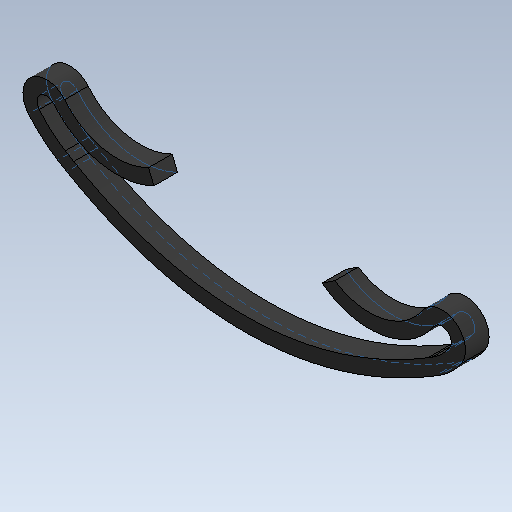
# Autodesk Inventor part: 脚ゴム
Saved by Autodesk Inventor 2020 (Build 240168000, 168)
## iProperties
Created: 2020-11-29
Part Number: 脚ゴム
Material: ゴム、黒
Document SubType Name: Modeling
Designer: AA19065
Density: 0.93 g/cm^3
Appearance: ゴム - 黒
Mass: 2.30491 g
Surface Area: 26.747 cm^2
Volume: 2.47839 cm^3
Author: AA19065
Autodesk Inventor part; units mm, degrees
ref_plane "YZ Plane" through (0, 0, 0) normal (1, 0, 0) x (0, 1, 0)
ref_plane "XZ Plane" through (0, 0, 0) normal (0, 1, 0) x (-1, 0, 0)
ref_plane "XY Plane" through (0, 0, 0) normal (0, 0, 1) x (1, 0, 0)
sketch "スケッチ1" plane through (0, 0, 0) normal (0, 0, 1) x (1, 0, 0)
  spline S0 degree 4 poles (38.5164, -45.3071) (32.8487, -48.7376) (24.871, -52.6644) (14.1977, -56.036) (0.8351, -57.2731) (-12.4819, -56.5781) (-23.1394, -53.6461) (-31.0456, -50.0372) (-36.604, -46.8264) knots 0 0 0 0 0 0.316482 0.440352 0.563601 0.687002 1 1 1 1 1
  circle A0 centre (0, 0) radius 1.3
  circle A1 centre (0, 0) radius 2.5
  circle A2 centre (0, 0) radius 5
  line L0 (4.899, 1) -> (9.798, -23)
  line L1 (-4.899, 1) -> (-9.798, -23)
  line L2 (-3.817, -10.1196) -> (-8.9705, -20.5808)
  circle A3 centre (0, -12) radius 4.255
  line L3 (3.817, -10.1196) -> (8.9705, -20.5808)
  circle A4 centre (0.0033, -24.9496) radius 10
  circle A5 centre (0, -25) radius 7.025
  spline S1 degree 4 poles (51.4895, -34.9586) (51.1529, -35.2256) (50.6846, -35.5944) (50.0873, -36.0604) (49.3638, -36.6179) (48.8453, -37.0139) (48.332, -37.4027) (47.8236, -37.7843) (47.3201, -38.159) (46.8211, -38.527) (46.3265, -38.8884) (45.8362, -39.2435) (45.3499, -39.5924) (44.8675, -39.9354) (44.3888, -40.2724) (43.9136, -40.6038) (43.4419, -40.9296) (42.9735, -41.25) (42.5081, -41.5651) (42.0458, -41.8751) (41.5864, -42.18) (41.1297, -42.48) (40.6756, -42.7752) (40.2241, -43.0657) (39.7749, -43.3517) (39.328, -43.6331) (38.8834, -43.9101) (38.4408, -44.1828) (38.0002, -44.4513) (37.5615, -44.7157) (37.1246, -44.9759) (36.6894, -45.2322) (36.2559, -45.4846) (35.8239, -45.7332) (35.3934, -45.9779) (34.9643, -46.2189) (34.5365, -46.4563) (34.1101, -46.6901) (33.6848, -46.9203) (33.2606, -47.1471) (32.8375, -47.3704) (32.4155, -47.5903) (31.9943, -47.8068) (31.5741, -48.0201) (31.1548, -48.23) (30.7362, -48.4368) (30.3184, -48.6403) (29.9013, -48.8407) (29.4848, -49.038) (29.069, -49.2322) (28.6537, -49.4233) (28.239, -49.6114) (27.8248, -49.7965) (27.411, -49.9786) (26.9977, -50.1578) (26.5847, -50.334) (26.1721, -50.5073) (25.7598, -50.6777) (25.3479, -50.8453) (24.9362, -51.01) (24.5247, -51.1719) (24.1135, -51.331) (23.7024, -51.4873) (23.2916, -51.6408) (22.8809, -51.7915) (22.4703, -51.9394) (22.0598, -52.0847) (21.6495, -52.2271) (21.2392, -52.3669) (20.829, -52.504) (20.4188, -52.6383) (20.0086, -52.77) (19.5985, -52.8989) (19.1884, -53.0252) (18.7783, -53.1489) (18.3681, -53.2698) (17.958, -53.3881) (17.5477, -53.5038) (17.1375, -53.6167) (16.7272, -53.7271) (16.3168, -53.8348) (15.9064, -53.9399) (15.4959, -54.0424) (15.0853, -54.1422) (14.6747, -54.2394) (14.2639, -54.334) (13.8531, -54.426) (13.4422, -54.5153) (13.0311, -54.6021) (12.62, -54.6862) (12.2088, -54.7677) (11.7975, -54.8466) (11.3861, -54.9229) (10.9746, -54.9966) (10.563, -55.0677) (10.1513, -55.1362) (9.7395, -55.2021) (9.3276, -55.2654) (8.9156, -55.3261) (8.5036, -55.3842) (8.0914, -55.4397) (7.6792, -55.4926) (7.2669, -55.5428) (6.8545, -55.5905) (6.4421, -55.6356) (6.0295, -55.6781) (5.617, -55.718) (5.2043, -55.7553) (4.7916, -55.79) (4.3789, -55.822) (3.9661, -55.8515) (3.5533, -55.8784) (3.1405, -55.9027) (2.7276, -55.9244) (2.3147, -55.9435) (1.9018, -55.96) (1.489, -55.9739) (1.0761, -55.9851) (0.6632, -55.9938) (0.2503, -55.9999) (-0.1625, -56.0034) (-0.5753, -56.0043) (-0.9881, -56.0026) (-1.4008, -55.9982) (-1.8134, -55.9913) (-2.2261, -55.9818) (-2.6386, -55.9697) (-3.0511, -55.955) (-3.4634, -55.9376) (-3.8757, -55.9177) (-4.2879, -55.8952) (-4.7, -55.8701) (-5.112, -55.8424) (-5.5239, -55.8121) (-5.9357, -55.7791) (-6.3473, -55.7436) (-6.7588, -55.7055) (-7.1701, -55.6648) (-7.5813, -55.6215) (-7.9923, -55.5756) (-8.4032, -55.5271) (-8.8139, -55.4761) (-9.2244, -55.4224) (-9.6348, -55.3661) (-10.0449, -55.3072) (-10.4549, -55.2458) (-10.8647, -55.1817) (-11.2743, -55.1151) (-11.6837, -55.0458) (-12.0928, -54.974) (-12.5018, -54.8995) (-12.9105, -54.8225) (-13.3191, -54.7429) (-13.7274, -54.6607) (-14.1355, -54.5759) (-14.5434, -54.4884) (-14.951, -54.3984) (-15.3585, -54.3058) (-15.7657, -54.2106) (-16.1727, -54.1128) (-16.5794, -54.0124) (-16.986, -53.9094) (-17.3923, -53.8038) (-17.7984, -53.6956) (-18.2043, -53.5848) (-18.61, -53.4713) (-19.0155, -53.3553) (-19.4208, -53.2366) (-19.8259, -53.1153) (-20.2308, -52.9913) (-20.6356, -52.8648) (-21.0401, -52.7355) (-21.4446, -52.6037) (-21.8489, -52.4692) (-22.253, -52.332) (-22.657, -52.1921) (-23.0609, -52.0496) (-23.4648, -51.9044) (-23.8685, -51.7565) (-24.2722, -51.6059) (-24.6759, -51.4526) (-25.0796, -51.2965) (-25.4832, -51.1377) (-25.8869, -50.9761) (-26.2907, -50.8117) (-26.6945, -50.6446) (-27.0985, -50.4746) (-27.5026, -50.3018) (-27.9068, -50.1261) (-28.3113, -49.9476) (-28.7161, -49.7661) (-29.1211, -49.5817) (-29.5265, -49.3944) (-29.9322, -49.204) (-30.3384, -49.0107) (-30.7451, -48.8142) (-31.1523, -48.6147) (-31.5601, -48.412) (-31.9685, -48.2062) (-32.3777, -47.9971) (-32.7876, -47.7847) (-33.1984, -47.569) (-33.6102, -47.3499) (-34.023, -47.1273) (-34.4368, -46.9012) (-34.8519, -46.6716) (-35.2682, -46.4382) (-35.686, -46.2011) (-36.1052, -45.9602) (-36.5261, -45.7154) (-36.9487, -45.4665) (-37.3732, -45.2135) (-37.7997, -44.9563) (-38.2284, -44.6947) (-38.6594, -44.4287) (-39.0929, -44.158) (-39.5291, -43.8825) (-39.9681, -43.6021) (-40.4101, -43.3165) (-40.8555, -43.0257) (-41.3043, -42.7295) (-41.7569, -42.4275) (-42.2135, -42.1196) (-42.6743, -41.8055) (-43.1398, -41.485) (-43.6102, -41.1578) (-44.0858, -40.8236) (-44.567, -40.482) (-45.0542, -40.1327) (-45.5479, -39.7753) (-46.0484, -39.4095) (-46.5564, -39.0347) (-47.0722, -38.6504) (-47.5966, -38.2562) (-48.13, -37.8515) (-48.6732, -37.4356) (-49.2269, -37.0078) (-50.01, -36.3976) (-50.6631, -35.8819) (-51.1798, -35.4699) (-51.5542, -35.1694) knots 0 0 0 0 0 0.01253 0.017489 0.022414 0.027307 0.032168 0.036998 0.041798 0.046569 0.051311 0.056026 0.060715 0.065378 0.070016 0.074629 0.079219 0.083786 0.088331 0.092854 0.097357 0.101839 0.106302 0.110746 0.115172 0.119579 0.12397 0.128343 0.132701 0.137042 0.141369 0.14568 0.149978 0.154261 0.158531 0.162788 0.167033 0.171265 0.175486 0.179695 0.183893 0.18808 0.192257 0.196424 0.200581 0.204729 0.208867 0.212997 0.217119 0.221232 0.225337 0.229434 0.233524 0.237607 0.241682 0.245751 0.249814 0.25387 0.25792 0.261964 0.266002 0.270035 0.274062 0.278085 0.282102 0.286114 0.290122 0.294125 0.298124 0.302119 0.30611 0.310097 0.31408 0.318059 0.322035 0.326007 0.329976 0.333942 0.337905 0.341865 0.345823 0.349777 0.353729 0.357678 0.361625 0.365569 0.369511 0.373451 0.377389 0.381325 0.385259 0.389191 0.393122 0.39705 0.400977 0.404903 0.408826 0.412749 0.41667 0.42059 0.424508 0.428426 0.432342 0.436257 0.440171 0.444085 0.447997 0.451908 0.455819 0.459729 0.463638 0.467547 0.471454 0.475362 0.479269 0.483175 0.487081 0.490987 0.494892 0.498797 0.502702 0.506607 0.510511 0.514415 0.51832 0.522224 0.526128 0.530033 0.533937 0.537842 0.541747 0.545652 0.549557 0.553463 0.557369 0.561276 0.565183 0.56909 0.572998 0.576907 0.580817 0.584727 0.588638 0.592549 0.596462 0.600375 0.60429 0.608205 0.612122 0.616039 0.619958 0.623879 0.6278 0.631723 0.635647 0.639573 0.643501 0.64743 0.651361 0.655294 0.659229 0.663165 0.667104 0.671045 0.674989 0.678934 0.682883 0.686833 0.690787 0.694743 0.698702 0.702664 0.70663 0.710598 0.71457 0.718546 0.722525 0.726508 0.730496 0.734487 0.738483 0.742483 0.746488 0.750498 0.754514 0.758534 0.76256 0.766592 0.77063 0.774674 0.778725 0.782783 0.786848 0.79092 0.795001 0.799089 0.803186 0.807291 0.811406 0.815531 0.819665 0.82381 0.827967 0.832134 0.836314 0.840506 0.844711 0.84893 0.853163 0.857412 0.861676 0.865957 0.870254 0.87457 0.878905 0.88326 0.887636 0.892033 0.896453 0.900898 0.905368 0.909864 0.914388 0.918942 0.923526 0.928143 0.932794 0.937481 0.942205 0.94697 0.951777 0.956628 0.961526 0.966473 0.971473 0.976527 0.981641 0.986815 1 1 1 1 1 construction
  line L4 (-36.604, -46.8264) -> (0, 0) construction
  line L5 (0, 0) -> (38.5164, -45.3071) construction
  line L6 (-38.4038, -45.7442) -> (0, 0) construction
  line L7 (39.4123, -44.7541) -> (0, 0) construction
  line L8 (0, 0) -> (-43.9228, -40.9378) construction
  line L9 (43.1454, -41.1321) -> (0, 0) construction
  arc A6 (-38.4038, -45.7442) -> (-36.604, -46.8264) centre (-6.5918, 5.1281) ccw
  arc A7 (38.5164, -45.3071) -> (39.4123, -44.7541) centre (7.4479, 6.0227) ccw
  arc A8 (-43.9228, -40.9378) -> (-38.4038, -45.7442) centre (-26.0471, -25.9839) ccw
  arc A9 (39.4123, -44.7541) -> (43.1454, -41.1321) centre (32.7173, -34.1188) ccw
  line L10 (36.2541, -30.9682) -> (42.4664, -35.652)
  line L11 (-31.1512, -26.4822) -> (-36.604, -31.0671)
  line L12 (-36.604, -96) -> (31.1535, -96) construction
  line L13 (-33.8776, -60) -> (44.0237, -60) construction
  line L14 (59.4013, -96) -> (59.4013, -81)
  line L15 (59.4013, -81) -> (-53.0814, -81) construction
  arc A10 (36.2232, -74.5536) -> (59.4013, -81) centre (70, 2) ccw construction
  line L16 (70, 2) -> (36.2232, -74.5536) construction
  line L17 (70, 2) -> (59.4013, -81) construction
  arc A11 (-71.6102, -42.5485) -> (-53.0814, -81) centre (70, 2) ccw construction
  line L18 (70, 2) -> (-71.6102, -42.5485) construction
  line L19 (70, 2) -> (-53.0814, -81) construction
  line L20 (-71.6102, -42.5485) -> (36.2232, -74.5536) construction
  arc A12 (-53.0814, -81) -> (-15.0732, -119.6576) centre (70, 2) ccw construction
  line L21 (70, 2) -> (-15.0732, -119.6576) construction
  line L22 (70, 2) -> (-53.0814, -81) construction
  arc A13 (59.4013, -81) -> (89.9091, -79.2709) centre (70, 2) ccw construction
  line L23 (70, 2) -> (89.9091, -79.2709) construction
  line L24 (70, 2) -> (59.4013, -81) construction
  line L25 (-15.0732, -119.6576) -> (89.9091, -79.2709) construction
  arc A14 (-40.8548, -38.3712) -> (-43.9228, -40.9378) centre (-42.3888, -39.6545) ccw
  line L26 (-43.9228, -40.9378) -> (-42.3888, -39.6545) construction
  line L27 (-40.8548, -38.3712) -> (-42.3888, -39.6545) construction
  arc A15 (43.1454, -41.1321) -> (39.8262, -38.8998) centre (41.4858, -40.016) ccw
  line L28 (43.1454, -41.1321) -> (41.4858, -40.016) construction
  line L29 (39.8262, -38.8998) -> (41.4858, -40.016) construction
  arc A16 (9.8434, -26.7306) -> (39.8262, -38.8998) centre (26.1095, -29.6747) ccw
  arc A17 (-40.8548, -38.3712) -> (-9.9651, -25.7437) centre (-27.4224, -27.1344) ccw
  arc A18 (-38.5537, -36.4463) -> (-12.9543, -25.9986) centre (-27.4224, -27.1344) ccw
  arc A19 (-38.5537, -36.4463) -> (-46.2238, -42.8627) centre (-42.3888, -39.6545) ccw
  arc A20 (-46.2238, -42.8627) -> (-39.9944, -48.2878) centre (-26.0471, -25.9839) ccw
  arc A21 (-39.9944, -48.2878) -> (-38.1046, -49.4241) centre (-6.5918, 5.1281) ccw
  arc A22 (40.0699, -47.8736) -> (41.0105, -47.2929) centre (7.4479, 6.0227) ccw
  arc A23 (41.0105, -47.2929) -> (45.6348, -42.8063) centre (32.7173, -34.1188) ccw
  arc A24 (45.6348, -42.8063) -> (37.3369, -37.2256) centre (41.4858, -40.016) ccw
  arc A25 (12.7927, -27.28) -> (37.3369, -37.2256) centre (26.1095, -29.6747) ccw
  line L30 (-20.7448, -40.0195) -> (-19.6157, -42.8107)
  line L31 (18.7559, -41.0323) -> (16.0741, -42.8103)
  spline S2 degree 4 poles (38.5164, -45.3071) (32.8478, -48.7393) (24.8691, -52.6682) (14.1948, -56.0416) (0.8318, -57.2787) (-12.4847, -56.5826) (-23.1412, -53.6487) (-31.0464, -50.0382) (-36.604, -46.8264) knots 0 0 0 0 0 0.316504 0.440374 0.56362 0.687015 1 1 1 1 1
  circle A26 centre (0, 0) radius 1.3
  circle A27 centre (0, 0) radius 2.5
  circle A28 centre (0, 0) radius 5
  line L32 (4.899, 1) -> (9.798, -23)
  line L33 (-4.899, 1) -> (-9.798, -23)
  line L34 (-3.817, -10.1196) -> (-8.9705, -20.5808)
  circle A29 centre (0, -12) radius 4.255
  line L35 (3.817, -10.1196) -> (8.9705, -20.5808)
  circle A30 centre (0.0012, -24.9711) radius 10
  circle A31 centre (0, -25) radius 7.025
  spline S3 degree 4 poles (51.4895, -34.9586) (51.1529, -35.2256) (50.6846, -35.5944) (50.0873, -36.0604) (49.3638, -36.6179) (48.8453, -37.0139) (48.332, -37.4027) (47.8236, -37.7843) (47.3201, -38.159) (46.8211, -38.527) (46.3265, -38.8884) (45.8362, -39.2435) (45.3499, -39.5924) (44.8675, -39.9354) (44.3888, -40.2724) (43.9136, -40.6038) (43.4419, -40.9296) (42.9735, -41.25) (42.5081, -41.5651) (42.0458, -41.8751) (41.5864, -42.18) (41.1297, -42.48) (40.6756, -42.7752) (40.2241, -43.0657) (39.7749, -43.3517) (39.328, -43.6331) (38.8834, -43.9101) (38.4408, -44.1828) (38.0002, -44.4513) (37.5615, -44.7157) (37.1246, -44.9759) (36.6894, -45.2322) (36.2559, -45.4846) (35.8239, -45.7332) (35.3934, -45.9779) (34.9643, -46.2189) (34.5365, -46.4563) (34.1101, -46.6901) (33.6848, -46.9203) (33.2606, -47.1471) (32.8375, -47.3704) (32.4155, -47.5903) (31.9943, -47.8068) (31.5741, -48.0201) (31.1548, -48.23) (30.7362, -48.4368) (30.3184, -48.6403) (29.9013, -48.8407) (29.4848, -49.038) (29.069, -49.2322) (28.6537, -49.4233) (28.239, -49.6114) (27.8248, -49.7965) (27.411, -49.9786) (26.9977, -50.1578) (26.5847, -50.334) (26.1721, -50.5073) (25.7598, -50.6777) (25.3479, -50.8453) (24.9362, -51.01) (24.5247, -51.1719) (24.1135, -51.331) (23.7024, -51.4873) (23.2916, -51.6408) (22.8809, -51.7915) (22.4703, -51.9394) (22.0598, -52.0847) (21.6495, -52.2271) (21.2392, -52.3669) (20.829, -52.504) (20.4188, -52.6383) (20.0086, -52.77) (19.5985, -52.8989) (19.1884, -53.0252) (18.7783, -53.1489) (18.3681, -53.2698) (17.958, -53.3881) (17.5477, -53.5038) (17.1375, -53.6167) (16.7272, -53.7271) (16.3168, -53.8348) (15.9064, -53.9399) (15.4959, -54.0424) (15.0853, -54.1422) (14.6747, -54.2394) (14.2639, -54.334) (13.8531, -54.426) (13.4422, -54.5153) (13.0311, -54.6021) (12.62, -54.6862) (12.2088, -54.7677) (11.7975, -54.8466) (11.3861, -54.9229) (10.9746, -54.9966) (10.563, -55.0677) (10.1513, -55.1362) (9.7395, -55.2021) (9.3276, -55.2654) (8.9156, -55.3261) (8.5036, -55.3842) (8.0914, -55.4397) (7.6792, -55.4926) (7.2669, -55.5428) (6.8545, -55.5905) (6.4421, -55.6356) (6.0295, -55.6781) (5.617, -55.718) (5.2043, -55.7553) (4.7916, -55.79) (4.3789, -55.822) (3.9661, -55.8515) (3.5533, -55.8784) (3.1405, -55.9027) (2.7276, -55.9244) (2.3147, -55.9435) (1.9018, -55.96) (1.489, -55.9739) (1.0761, -55.9851) (0.6632, -55.9938) (0.2503, -55.9999) (-0.1625, -56.0034) (-0.5753, -56.0043) (-0.9881, -56.0026) (-1.4008, -55.9982) (-1.8134, -55.9913) (-2.2261, -55.9818) (-2.6386, -55.9697) (-3.0511, -55.955) (-3.4634, -55.9376) (-3.8757, -55.9177) (-4.2879, -55.8952) (-4.7, -55.8701) (-5.112, -55.8424) (-5.5239, -55.8121) (-5.9357, -55.7791) (-6.3473, -55.7436) (-6.7588, -55.7055) (-7.1701, -55.6648) (-7.5813, -55.6215) (-7.9923, -55.5756) (-8.4032, -55.5271) (-8.8139, -55.4761) (-9.2244, -55.4224) (-9.6348, -55.3661) (-10.0449, -55.3072) (-10.4549, -55.2458) (-10.8647, -55.1817) (-11.2743, -55.1151) (-11.6837, -55.0458) (-12.0928, -54.974) (-12.5018, -54.8995) (-12.9105, -54.8225) (-13.3191, -54.7429) (-13.7274, -54.6607) (-14.1355, -54.5759) (-14.5434, -54.4884) (-14.951, -54.3984) (-15.3585, -54.3058) (-15.7657, -54.2106) (-16.1727, -54.1128) (-16.5794, -54.0124) (-16.986, -53.9094) (-17.3923, -53.8038) (-17.7984, -53.6956) (-18.2043, -53.5848) (-18.61, -53.4713) (-19.0155, -53.3553) (-19.4208, -53.2366) (-19.8259, -53.1153) (-20.2308, -52.9913) (-20.6356, -52.8648) (-21.0401, -52.7355) (-21.4446, -52.6037) (-21.8489, -52.4692) (-22.253, -52.332) (-22.657, -52.1921) (-23.0609, -52.0496) (-23.4648, -51.9044) (-23.8685, -51.7565) (-24.2722, -51.6059) (-24.6759, -51.4526) (-25.0796, -51.2965) (-25.4832, -51.1377) (-25.8869, -50.9761) (-26.2907, -50.8117) (-26.6945, -50.6446) (-27.0985, -50.4746) (-27.5026, -50.3018) (-27.9068, -50.1261) (-28.3113, -49.9476) (-28.7161, -49.7661) (-29.1211, -49.5817) (-29.5265, -49.3944) (-29.9322, -49.204) (-30.3384, -49.0107) (-30.7451, -48.8142) (-31.1523, -48.6147) (-31.5601, -48.412) (-31.9685, -48.2062) (-32.3777, -47.9971) (-32.7876, -47.7847) (-33.1984, -47.569) (-33.6102, -47.3499) (-34.023, -47.1273) (-34.4368, -46.9012) (-34.8519, -46.6716) (-35.2682, -46.4382) (-35.686, -46.2011) (-36.1052, -45.9602) (-36.5261, -45.7154) (-36.9487, -45.4665) (-37.3732, -45.2135) (-37.7997, -44.9563) (-38.2284, -44.6947) (-38.6594, -44.4287) (-39.0929, -44.158) (-39.5291, -43.8825) (-39.9681, -43.6021) (-40.4101, -43.3165) (-40.8555, -43.0257) (-41.3043, -42.7295) (-41.7569, -42.4275) (-42.2135, -42.1196) (-42.6743, -41.8055) (-43.1398, -41.485) (-43.6102, -41.1578) (-44.0858, -40.8236) (-44.567, -40.482) (-45.0542, -40.1327) (-45.5479, -39.7753) (-46.0484, -39.4095) (-46.5564, -39.0347) (-47.0722, -38.6504) (-47.5966, -38.2562) (-48.13, -37.8515) (-48.6732, -37.4356) (-49.2269, -37.0078) (-50.01, -36.3976) (-50.6631, -35.8819) (-51.1798, -35.4699) (-51.5542, -35.1694) knots 0 0 0 0 0 0.01253 0.017489 0.022414 0.027307 0.032168 0.036998 0.041798 0.046569 0.051311 0.056026 0.060715 0.065378 0.070016 0.074629 0.079219 0.083786 0.088331 0.092854 0.097357 0.101839 0.106302 0.110746 0.115172 0.119579 0.12397 0.128343 0.132701 0.137042 0.141369 0.14568 0.149978 0.154261 0.158531 0.162788 0.167033 0.171265 0.175486 0.179695 0.183893 0.18808 0.192257 0.196424 0.200581 0.204729 0.208867 0.212997 0.217119 0.221232 0.225337 0.229434 0.233524 0.237607 0.241682 0.245751 0.249814 0.25387 0.25792 0.261964 0.266002 0.270035 0.274062 0.278085 0.282102 0.286114 0.290122 0.294125 0.298124 0.302119 0.30611 0.310097 0.31408 0.318059 0.322035 0.326007 0.329976 0.333942 0.337905 0.341865 0.345823 0.349777 0.353729 0.357678 0.361625 0.365569 0.369511 0.373451 0.377389 0.381325 0.385259 0.389191 0.393122 0.39705 0.400977 0.404903 0.408826 0.412749 0.41667 0.42059 0.424508 0.428426 0.432342 0.436257 0.440171 0.444085 0.447997 0.451908 0.455819 0.459729 0.463638 0.467547 0.471454 0.475362 0.479269 0.483175 0.487081 0.490987 0.494892 0.498797 0.502702 0.506607 0.510511 0.514415 0.51832 0.522224 0.526128 0.530033 0.533937 0.537842 0.541747 0.545652 0.549557 0.553463 0.557369 0.561276 0.565183 0.56909 0.572998 0.576907 0.580817 0.584727 0.588638 0.592549 0.596462 0.600375 0.60429 0.608205 0.612122 0.616039 0.619958 0.623879 0.6278 0.631723 0.635647 0.639573 0.643501 0.64743 0.651361 0.655294 0.659229 0.663165 0.667104 0.671045 0.674989 0.678934 0.682883 0.686833 0.690787 0.694743 0.698702 0.702664 0.70663 0.710598 0.71457 0.718546 0.722525 0.726508 0.730496 0.734487 0.738483 0.742483 0.746488 0.750498 0.754514 0.758534 0.76256 0.766592 0.77063 0.774674 0.778725 0.782783 0.786848 0.79092 0.795001 0.799089 0.803186 0.807291 0.811406 0.815531 0.819665 0.82381 0.827967 0.832134 0.836314 0.840506 0.844711 0.84893 0.853163 0.857412 0.861676 0.865957 0.870254 0.87457 0.878905 0.88326 0.887636 0.892033 0.896453 0.900898 0.905368 0.909864 0.914388 0.918942 0.923526 0.928143 0.932794 0.937481 0.942205 0.94697 0.951777 0.956628 0.961526 0.966473 0.971473 0.976527 0.981641 0.986815 1 1 1 1 1 construction
  line L36 (-36.604, -46.8264) -> (0, 0) construction
  line L37 (0, 0) -> (38.5164, -45.3071) construction
  line L38 (-38.4035, -45.7439) -> (0, 0) construction
  line L39 (39.4122, -44.754) -> (0, 0) construction
  line L40 (0, 0) -> (-43.9228, -40.9378) construction
  line L41 (43.1454, -41.1321) -> (0, 0) construction
  arc A32 (-38.4035, -45.7439) -> (-36.604, -46.8264) centre (-6.5817, 5.1223) ccw
  arc A33 (38.5164, -45.3071) -> (39.4122, -44.754) centre (7.4403, 6.0181) ccw
  arc A34 (-43.9228, -40.9378) -> (-38.4035, -45.7439) centre (-26.0235, -25.9549) ccw
  arc A35 (39.4122, -44.754) -> (43.1454, -41.1321) centre (32.7099, -34.1106) ccw
  line L42 (36.2541, -30.9682) -> (42.4664, -35.652)
  line L43 (-31.1512, -26.4822) -> (-36.604, -31.0671)
  line L44 (-36.604, -96) -> (31.1535, -96) construction
  line L45 (-33.8776, -60) -> (44.0237, -60) construction
  line L46 (59.4013, -96) -> (59.4013, -81)
  line L47 (59.4013, -81) -> (-53.0814, -81) construction
  arc A36 (36.2232, -74.5536) -> (59.4013, -81) centre (70, 2) ccw construction
  line L48 (70, 2) -> (36.2232, -74.5536) construction
  line L49 (70, 2) -> (59.4013, -81) construction
  arc A37 (-71.6102, -42.5485) -> (-53.0814, -81) centre (70, 2) ccw construction
  line L50 (70, 2) -> (-71.6102, -42.5485) construction
  line L51 (70, 2) -> (-53.0814, -81) construction
  line L52 (-71.6102, -42.5485) -> (36.2232, -74.5536) construction
  arc A38 (-53.0814, -81) -> (-15.0732, -119.6576) centre (70, 2) ccw construction
  line L53 (70, 2) -> (-15.0732, -119.6576) construction
  line L54 (70, 2) -> (-53.0814, -81) construction
  arc A39 (59.4013, -81) -> (89.9091, -79.2709) centre (70, 2) ccw construction
  line L55 (70, 2) -> (89.9091, -79.2709) construction
  line L56 (70, 2) -> (59.4013, -81) construction
  line L57 (-15.0732, -119.6576) -> (89.9091, -79.2709) construction
  arc A40 (-40.8555, -38.3703) -> (-43.9228, -40.9378) centre (-42.3892, -39.654) ccw
  line L58 (-43.9228, -40.9378) -> (-42.3892, -39.654) construction
  line L59 (-40.8555, -38.3703) -> (-42.3892, -39.654) construction
  arc A41 (43.1454, -41.1321) -> (39.8267, -38.8991) centre (41.4861, -40.0156) ccw
  line L60 (43.1454, -41.1321) -> (41.4861, -40.0156) construction
  line L61 (39.8267, -38.8991) -> (41.4861, -40.0156) construction
  arc A42 (9.843, -26.7427) -> (39.8267, -38.8991) centre (26.1119, -29.6712) ccw
  arc A43 (-40.8555, -38.3703) -> (-9.968, -25.7556) centre (-27.4267, -27.1294) ccw
  spline S4 degree 5 poles (-38.1046, -49.4241) (-30.9925, -53.5325) (-23.4374, -56.8772) (-15.4062, -59.1353) (1.1247, -61.1969) (17.5495, -58.3842) (25.5171, -55.7659) (32.9958, -52.1545) (40.0699, -47.8736) knots 0 0 0 0 0 0 0.498337 0.498337 0.498337 1 1 1 1 1 1
  point P0 (50.9482, -35.3862)
  point P1 (50.4129, -35.8055)
  point P2 (49.8835, -36.2167)
  point P3 (49.3597, -36.6202)
  point P4 (48.8414, -37.0162)
  point P5 (48.3282, -37.4048)
  point P6 (47.82, -37.7863)
  point P7 (47.3165, -38.1609)
  point P8 (46.8177, -38.5288)
  point P9 (46.3232, -38.8901)
  point P10 (45.833, -39.2452)
  point P11 (45.3467, -39.594)
  point P12 (44.8644, -39.9368)
  point P13 (44.3858, -40.2738)
  point P14 (43.9108, -40.6051)
  point P15 (43.4391, -40.9309)
  point P16 (42.9708, -41.2512)
  point P17 (42.5055, -41.5662)
  point P18 (42.0433, -41.8761)
  point P19 (41.5839, -42.181)
  point P20 (41.1273, -42.4809)
  point P21 (40.6733, -42.7761)
  point P22 (40.2218, -43.0666)
  point P23 (39.7727, -43.3524)
  point P24 (39.3259, -43.6338)
  point P25 (38.8813, -43.9108)
  point P26 (38.4387, -44.1834)
  point P27 (37.9982, -44.4519)
  point P28 (37.5596, -44.7162)
  point P29 (37.1227, -44.9764)
  point P30 (36.6876, -45.2327)
  point P31 (36.2541, -45.485)
  point P32 (35.8222, -45.7335)
  point P33 (35.3917, -45.9782)
  point P34 (34.9627, -46.2192)
  point P35 (34.535, -46.4566)
  point P36 (34.1085, -46.6903)
  point P37 (33.6833, -46.9205)
  point P38 (33.2592, -47.1472)
  point P39 (32.8361, -47.3705)
  point P40 (32.4141, -47.5904)
  point P41 (31.993, -47.8069)
  point P42 (31.5729, -48.0201)
  point P43 (31.1535, -48.23)
  point P44 (30.735, -48.4368)
  point P45 (30.3172, -48.6403)
  point P46 (29.9002, -48.8407)
  point P47 (29.4837, -49.0379)
  point P48 (29.0679, -49.2321)
  point P49 (28.6527, -49.4232)
  point P50 (28.238, -49.6113)
  point P51 (27.8238, -49.7963)
  point P52 (27.41, -49.9784)
  point P53 (26.9967, -50.1576)
  point P54 (26.5838, -50.3338)
  point P55 (26.1712, -50.5071)
  point P56 (25.759, -50.6775)
  point P57 (25.347, -50.8451)
  point P58 (24.9353, -51.0098)
  point P59 (24.5239, -51.1717)
  point P60 (24.1127, -51.3307)
  point P61 (23.7017, -51.487)
  point P62 (23.2909, -51.6405)
  point P63 (22.8802, -51.7912)
  point P64 (22.4696, -51.9391)
  point P65 (22.0592, -52.0843)
  point P66 (21.6488, -52.2268)
  point P67 (21.2386, -52.3666)
  point P68 (20.8284, -52.5036)
  point P69 (20.4182, -52.6379)
  point P70 (20.0081, -52.7696)
  point P71 (19.598, -52.8986)
  point P72 (19.1879, -53.0248)
  point P73 (18.7777, -53.1485)
  point P74 (18.3676, -53.2694)
  point P75 (17.9575, -53.3877)
  point P76 (17.5473, -53.5033)
  point P77 (17.137, -53.6163)
  point P78 (16.7267, -53.7267)
  point P79 (16.3164, -53.8344)
  point P80 (15.906, -53.9395)
  point P81 (15.4955, -54.0419)
  point P82 (15.0849, -54.1417)
  point P83 (14.6743, -54.2389)
  point P84 (14.2635, -54.3335)
  point P85 (13.8527, -54.4255)
  point P86 (13.4418, -54.5148)
  point P87 (13.0308, -54.6016)
  point P88 (12.6197, -54.6857)
  point P89 (12.2085, -54.7672)
  point P90 (11.7972, -54.8461)
  point P91 (11.3858, -54.9224)
  point P92 (10.9743, -54.9961)
  point P93 (10.5627, -55.0672)
  point P94 (10.151, -55.1357)
  point P95 (9.7393, -55.2016)
  point P96 (9.3274, -55.2649)
  point P97 (8.9154, -55.3256)
  point P98 (8.5034, -55.3837)
  point P99 (8.0912, -55.4391)
  point P100 (7.679, -55.492)
  point P101 (7.2667, -55.5423)
  point P102 (6.8543, -55.59)
  point P103 (6.4419, -55.6351)
  point P104 (6.0294, -55.6776)
  point P105 (5.6168, -55.7175)
  point P106 (5.2042, -55.7547)
  point P107 (4.7915, -55.7894)
  point P108 (4.3788, -55.8215)
  point P109 (3.966, -55.851)
  point P110 (3.5532, -55.8779)
  point P111 (3.1404, -55.9022)
  point P112 (2.7275, -55.9239)
  point P113 (2.3147, -55.9429)
  point P114 (1.9018, -55.9594)
  point P115 (1.4889, -55.9733)
  point P116 (1.076, -55.9846)
  point P117 (0.6632, -55.9933)
  point P118 (0.2503, -55.9994)
  point P119 (-0.1625, -56.0028)
  point P120 (-0.5753, -56.0037)
  point P121 (-0.9881, -56.002)
  point P122 (-1.4008, -55.9977)
  point P123 (-1.8134, -55.9908)
  point P124 (-2.226, -55.9813)
  point P125 (-2.6386, -55.9691)
  point P126 (-3.051, -55.9544)
  point P127 (-3.4634, -55.9371)
  point P128 (-3.8757, -55.9172)
  point P129 (-4.2879, -55.8947)
  point P130 (-4.7, -55.8695)
  point P131 (-5.112, -55.8418)
  point P132 (-5.5238, -55.8115)
  point P133 (-5.9356, -55.7786)
  point P134 (-6.3472, -55.7431)
  point P135 (-6.7586, -55.705)
  point P136 (-7.17, -55.6643)
  point P137 (-7.5812, -55.621)
  point P138 (-7.9922, -55.5751)
  point P139 (-8.403, -55.5266)
  point P140 (-8.8137, -55.4755)
  point P141 (-9.2243, -55.4219)
  point P142 (-9.6346, -55.3656)
  point P143 (-10.0447, -55.3067)
  point P144 (-10.4547, -55.2452)
  point P145 (-10.8645, -55.1812)
  point P146 (-11.2741, -55.1145)
  point P147 (-11.6834, -55.0453)
  point P148 (-12.0926, -54.9735)
  point P149 (-12.5016, -54.899)
  point P150 (-12.9103, -54.822)
  point P151 (-13.3188, -54.7424)
  point P152 (-13.7271, -54.6602)
  point P153 (-14.1352, -54.5754)
  point P154 (-14.5431, -54.488)
  point P155 (-14.9507, -54.398)
  point P156 (-15.3582, -54.3054)
  point P157 (-15.7654, -54.2102)
  point P158 (-16.1723, -54.1124)
  point P159 (-16.5791, -54.012)
  point P160 (-16.9856, -53.909)
  point P161 (-17.3919, -53.8034)
  point P162 (-17.798, -53.6951)
  point P163 (-18.2039, -53.5843)
  point P164 (-18.6096, -53.4709)
  point P165 (-19.0151, -53.3548)
  point P166 (-19.4204, -53.2361)
  point P167 (-19.8255, -53.1148)
  point P168 (-20.2304, -52.9909)
  point P169 (-20.6351, -52.8643)
  point P170 (-21.0397, -52.7351)
  point P171 (-21.4441, -52.6033)
  point P172 (-21.8483, -52.4688)
  point P173 (-22.2525, -52.3316)
  point P174 (-22.6565, -52.1918)
  point P175 (-23.0604, -52.0493)
  point P176 (-23.4642, -51.9041)
  point P177 (-23.8679, -51.7562)
  point P178 (-24.2716, -51.6056)
  point P179 (-24.6752, -51.4522)
  point P180 (-25.0789, -51.2962)
  point P181 (-25.4825, -51.1374)
  point P182 (-25.8862, -50.9758)
  point P183 (-26.2899, -50.8115)
  point P184 (-26.6937, -50.6443)
  point P185 (-27.0977, -50.4744)
  point P186 (-27.5017, -50.3016)
  point P187 (-27.906, -50.1259)
  point P188 (-28.3104, -49.9474)
  point P189 (-28.7152, -49.766)
  point P190 (-29.1202, -49.5816)
  point P191 (-29.5255, -49.3943)
  point P192 (-29.9312, -49.2039)
  point P193 (-30.3374, -49.0106)
  point P194 (-30.744, -48.8142)
  point P195 (-31.1512, -48.6147)
  point P196 (-31.5589, -48.412)
  point P197 (-31.9673, -48.2062)
  point P198 (-32.3764, -47.9971)
  point P199 (-32.7863, -47.7848)
  dimension "d0" = 2
  dimension "d1" = 1
  dimension "d2" = 7
  dimension "d3" = 5
  dimension "d4" = 60
  dimension "d5" = 60
  dimension "d6" = 96
  dimension "d7" = 60
  dimension "d8" = 36
  dimension "d9" = 15
  dimension "d10" = 90
  dimension "d11" = 15
  dimension "d12" = 16.531
  dimension "d13" = 16.531
  dimension "d14" = 21.042
  dimension "d15" = 21.042
  dimension "d16" = 2
  dimension "d17" = 180
  dimension "d18" = 2
  dimension "d19" = 180
  dimension "d20" = 16.5303
  dimension "d21" = 44.1339
  dimension "d22" = 18.5303
  dimension "d23" = 87.0684
  dimension "d29" = 3
  dimension "d32" = 2
  dimension "d33" = 1
  dimension "d34" = 7
  dimension "d35" = 5
  dimension "d36" = 60
  dimension "d37" = 60
  dimension "d38" = 96
  dimension "d39" = 60
  dimension "d40" = 36
  dimension "d41" = 15
  dimension "d42" = 90
  dimension "d43" = 15
  dimension "d44" = 16.531
  dimension "d45" = 16.531
  dimension "d46" = 21.042
  dimension "d47" = 21.042
  dimension "d48" = 2
  dimension "d49" = 180
  dimension "d50" = 2
  dimension "d51" = 180
  dimension "d52" = 16.5303
  dimension "d53" = 44.1286
  dimension "d54" = 18.5303
  dimension "d55" = 87.0684
  constraints: 124 end point, 68 point on circle, 42 centre point, 12 tangent, 8 coincident, 4 horizontal, 2 concentric, 2 point on line, 2 vertical, 1011 other
  measures "d0" angle of L6 L4
  measures "d1" angle of L7 L5
  measures "d2" angle of L8 L6
  measures "d3" angle of L7 L9
  measures "d4" radius of A6
  measures "d5" radius of A7
  measures "d6" distance from line of L12 point (0, 0)
  measures "d7" distance from line of L13 point (0, 0)
  measures "d8" distance between parallel lines of L12 L13
  measures "d9" distance of L14.start L14.end
  measures "d10" angle of L15 L14
  measures "d11" distance from line of L12 L15.end
  measures "d12" angle of L16 L17
  measures "d13" angle of L18 L19
  measures "d14" angle of L22 L21
  measures "d15" angle of L24 L23
  measures "d16" radius of A14
  measures "d17" angle of L26 L27
  measures "d18" radius of A15
  measures "d19" angle of L28 L29
  measures "d20" radius of A16
  measures "d21" distance of point (0.003, -24.95) L28.end
  measures "d22" distance of L28.end A16.centre
  measures "d23" distance of L8.end L9.start
  measures "d29" radial gap between concentric circles of A17 A18
  measures "d32" angle of L38 L36
  measures "d33" angle of L39 L37
  measures "d34" angle of L40 L38
  measures "d35" angle of L39 L41
  measures "d36" radius of A32
  measures "d37" radius of A33
  measures "d38" distance from line of L44 point (0, 0)
  measures "d39" distance from line of L45 point (0, 0)
  measures "d40" distance between parallel lines of L44 L45
  measures "d41" distance of L46.start L46.end
  measures "d42" angle of L47 L46
  measures "d43" distance from line of L44 L47.end
  measures "d44" angle of L48 L49
  measures "d45" angle of L50 L51
  measures "d46" angle of L54 L53
  measures "d47" angle of L56 L55
  measures "d48" radius of A40
  measures "d49" angle of L58 L59
  measures "d50" radius of A41
  measures "d51" angle of L60 L61
  measures "d52" radius of A42
  measures "d53" distance of point (0.001, -24.971) L60.end
  measures "d54" distance of L60.end A42.centre
  measures "d55" distance of L40.end L41.start
extrude "押し出し1" add sketch "スケッチ1" along normal blind 5 contours A7 A9 A15 A16 L31 A25 A24 A23 A22 S4 A21 A20 A19 A18 L30 A43 A14 A8 A6 S2 | A43 L30 A17
equation "\"d6\" = d26 + d28 + d27"
equation "\"d7\" = d26 - d28 + d27"
equation "\"d11\" = d9"
equation "\"d12\" = d13"
equation "\"d13\" = d24"
equation "\"d14\" = d15"
equation "\"d15\" = d25"
equation "\"d38\" = d58 + d60 + d59"
equation "\"d39\" = d58 - d60 + d59"
equation "\"d43\" = d41"
equation "\"d44\" = d45"
equation "\"d45\" = d56"
equation "\"d46\" = d47"
equation "\"d47\" = d57"
equation "\"d24\" = 16.530955deg"
equation "\"d25\" = 21.041744deg"
equation "\"d56\" = 16.530955deg"
equation "\"d57\" = 21.041744deg"
equation "\"d26\" = 53"
equation "\"d28\" = 18"
equation "\"d27\" = 25"
equation "\"d58\" = 53"
equation "\"d60\" = 18"
equation "\"d59\" = 25"
